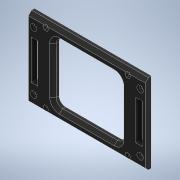
# Autodesk Inventor part: BottomHolder
Saved by Autodesk Inventor 2021 (Build 250183000, 183)
## iProperties
Created: 2020-11-06
Part Number: BottomHolder
Material: Generic
Document SubType Name: Modeling
Designer: lgnds
Density: 1 g/cm^3
Appearance: Default
Author: lgnds
Autodesk Inventor part; units mm, degrees
ref_plane "YZ Plane" through (0, 0, 0) normal (1, 0, 0) x (0, 1, 0)
ref_plane "XZ Plane" through (0, 0, 0) normal (0, 1, 0) x (-1, 0, 0)
ref_plane "XY Plane" through (0, 0, 0) normal (0, 0, 1) x (1, 0, 0)
sketch "Sketch1" plane through (0, 0, 0) normal (0, 0, 1) x (1, 0, 0)
  line L0 (-63.5, -54) -> (63.5, -54) construction
  line L1 (63.5, -54) -> (63.5, 54) construction
  line L2 (63.5, 54) -> (-63.5, 54) construction
  line L3 (-63.5, 54) -> (-63.5, -54) construction
  line L4 (-63.5, -54) -> (63.5, 54) construction
  line L5 (63.5, -54) -> (-63.5, 54) construction
  line L6 (-61.2483, 57.9) -> (-58.9967, 54) construction
  line L7 (-58.9967, 54) -> (-61.2483, 50.1) construction
  line L8 (-61.2483, 50.1) -> (-65.7517, 50.1) construction
  line L9 (-65.7517, 50.1) -> (-68.0033, 54) construction
  line L10 (-68.0033, 54) -> (-65.7517, 57.9) construction
  line L11 (-65.7517, 57.9) -> (-61.2483, 57.9) construction
  line L12 (-98.7, 0) -> (98.7, 0) construction
  line L13 (0, 86.8) -> (0, -86.8) construction
  line L14 (61.2483, 57.9) -> (58.9967, 54) construction
  line L15 (58.9967, 54) -> (61.2483, 50.1) construction
  line L16 (61.2483, 50.1) -> (65.7517, 50.1) construction
  line L17 (65.7517, 50.1) -> (68.0033, 54) construction
  line L18 (68.0033, 54) -> (65.7517, 57.9) construction
  line L19 (65.7517, 57.9) -> (61.2483, 57.9) construction
  line L20 (63.5, -54) -> (-63.5, -54) construction
  line L21 (-61.2483, -57.9) -> (-58.9967, -54) construction
  line L22 (-58.9967, -54) -> (-61.2483, -50.1) construction
  line L23 (-61.2483, -50.1) -> (-65.7517, -50.1) construction
  line L24 (-65.7517, -50.1) -> (-68.0033, -54) construction
  line L25 (-68.0033, -54) -> (-65.7517, -57.9) construction
  line L26 (-65.7517, -57.9) -> (-61.2483, -57.9) construction
  line L27 (61.2483, -57.9) -> (58.9967, -54) construction
  line L28 (58.9967, -54) -> (61.2483, -50.1) construction
  line L29 (61.2483, -50.1) -> (65.7517, -50.1) construction
  line L30 (65.7517, -50.1) -> (68.0033, -54) construction
  line L31 (68.0033, -54) -> (65.7517, -57.9) construction
  line L32 (65.7517, -57.9) -> (61.2483, -57.9) construction
  line L33 (-70.5, -62) -> (70.5, -62)
  line L34 (70.5, -62) -> (70.5, 62)
  line L35 (70.5, 62) -> (-70.5, 62)
  line L36 (-70.5, 62) -> (-70.5, -62)
  line L37 (-70.5, -62) -> (70.5, 62) construction
  line L38 (70.5, -62) -> (-70.5, 62) construction
  line L39 (-52.5, -46.1702) -> (52.5, -46.1702)
  line L40 (52.5, -46.1702) -> (52.5, 46.1702)
  line L41 (52.5, 46.1702) -> (-52.5, 46.1702)
  line L42 (-52.5, 46.1702) -> (-52.5, -46.1702)
  line L43 (-52.5, -46.1702) -> (52.5, 46.1702) construction
  line L44 (52.5, -46.1702) -> (-52.5, 46.1702) construction
  circle A0 centre (-63.5, 54) radius 2.4
  circle A1 centre (63.5, 54) radius 2.4
  circle A2 centre (63.5, -54) radius 2.4
  circle A3 centre (-63.5, -54) radius 2.4
  point P0 (0, 0)
  dimension "d0" = 7.8
  dimension "d1" = 127
  dimension "d2" = 108
  dimension "d3" = 124
  dimension "d4" = 141
  dimension "d5" = 18
  dimension "d8" = 4.8
  dimension "d9" = 4.8
  dimension "d10" = 4.8
  dimension "d11" = 4.8
  constraints: 86 end point, 21 symmetric about line, 8 coincident, 6 midpoint, 6 parallel, 4 centre point, 4 horizontal, 3 perpendicular, 1 point on line, 13 other
  measures "d0" distance between parallel lines of L8 L11
  measures "d1" distance of L1.end L2.end
  measures "d2" distance of L0.start L2.end
  measures "d3" distance between parallel lines of L33 L35
  measures "d4" distance between parallel lines of L34 L36
  measures "d5" distance between parallel lines of L36 L42
  measures "d8" diameter of A0
  measures "d9" diameter of A3
  measures "d10" diameter of A2
  measures "d11" diameter of A1
extrude "Extrusion1" add sketch "Sketch1" along normal blind 10
sketch "Sketch3" plane through (0, 0, 10) normal (0, 0, 1) x (1, 0, 0)
  circle A0 centre (-63.5, 54) radius 2.4 construction
  line L0 (-98.7, 0) -> (98.7, 0) construction
  line L1 (0, 86.8) -> (0, -86.8) construction
  line L2 (-61.2483, 57.9) -> (-58.9967, 54)
  line L3 (-58.9967, 54) -> (-61.2483, 50.1)
  line L4 (-61.2483, 50.1) -> (-65.7517, 50.1)
  line L5 (-65.7517, 50.1) -> (-68.0033, 54)
  line L6 (-68.0033, 54) -> (-65.7517, 57.9)
  line L7 (-65.7517, 57.9) -> (-61.2483, 57.9)
  circle A1 centre (63.5, 54) radius 2.4 construction
  line L8 (61.2483, 57.9) -> (58.9967, 54)
  line L9 (58.9967, 54) -> (61.2483, 50.1)
  line L10 (61.2483, 50.1) -> (65.7517, 50.1)
  line L11 (65.7517, 50.1) -> (68.0033, 54)
  line L12 (68.0033, 54) -> (65.7517, 57.9)
  line L13 (65.7517, 57.9) -> (61.2483, 57.9)
  circle A2 centre (-63.5, -54) radius 2.4 construction
  line L14 (-61.2483, -57.9) -> (-58.9967, -54)
  line L15 (-58.9967, -54) -> (-61.2483, -50.1)
  line L16 (-61.2483, -50.1) -> (-65.7517, -50.1)
  line L17 (-65.7517, -50.1) -> (-68.0033, -54)
  line L18 (-68.0033, -54) -> (-65.7517, -57.9)
  line L19 (-65.7517, -57.9) -> (-61.2483, -57.9)
  circle A3 centre (63.5, -54) radius 2.4 construction
  line L20 (61.2483, -57.9) -> (58.9967, -54)
  line L21 (58.9967, -54) -> (61.2483, -50.1)
  line L22 (61.2483, -50.1) -> (65.7517, -50.1)
  line L23 (65.7517, -50.1) -> (68.0033, -54)
  line L24 (68.0033, -54) -> (65.7517, -57.9)
  line L25 (65.7517, -57.9) -> (61.2483, -57.9)
  point P0 (0, 0)
  dimension "d12" = 7.8
  constraints: 48 end point, 24 symmetric about line, 4 coincident, 3 centre point, 1 horizontal, 16 other
  measures "d12" distance between parallel lines of L4 L7
extrude "Extrusion2" cut sketch "Sketch3" against normal blind 4
fillet "Fillet1" radius 10 4 edges at (-52.5, 46.1702, 5) (52.5, 46.1702, 5) (52.5, -46.1702, 5) (-52.5, -46.1702, 5)
chamfer "Chamfer1" distance 5 angle 45 8 edges at (0, 46.1702, 10) (49.5711, 43.2413, 10) (52.5, 0, 10) (49.5711, -43.2413, 10) (0, -46.1702, 10) (-49.5711, -43.2413, 10) (-52.5, 0, 10) (-49.5711, 43.2413, 10)
sketch "Sketch4" plane through (0, 0, 10) normal (0, 0, 1) x (1, 0, 0)
  line L0 (-70.5, -62) -> (70.5, -62) projected
  line L1 (-70.5, 62) -> (-90.5, 62)
  line L2 (-90.5, 62) -> (-90.5, -62)
  line L3 (-90.5, -62) -> (-70.5, -62)
  line L4 (-70.5, -62) -> (-70.5, 62)
  line L5 (0, 86.8) -> (0, -86.8) projected
  line L6 (70.5, 62) -> (90.5, 62)
  line L7 (90.5, 62) -> (90.5, -62)
  line L8 (90.5, -62) -> (70.5, -62)
  line L9 (70.5, -62) -> (70.5, 62)
  line L10 (-82.5, 62) -> (-82.5, -62) construction
  line L11 (-85.5, -30) -> (-79.5, -30)
  line L12 (-79.5, -30) -> (-79.5, 30)
  line L13 (-79.5, 30) -> (-85.5, 30)
  line L14 (-85.5, 30) -> (-85.5, -30)
  line L15 (-85.5, -30) -> (-79.5, 30) construction
  line L16 (-79.5, -30) -> (-85.5, 30) construction
  line L17 (82.5, 62) -> (82.5, -62) construction
  line L18 (85.5, -30) -> (79.5, -30)
  line L19 (79.5, -30) -> (79.5, 30)
  line L20 (79.5, 30) -> (85.5, 30)
  line L21 (85.5, 30) -> (85.5, -30)
  line L22 (85.5, -30) -> (79.5, 30) construction
  line L23 (79.5, -30) -> (85.5, 30) construction
  point P0 (0, 0)
  point P1 (-80.5, -62)
  point P2 (70.5, -62)
  point P3 (80.5, -62)
  point P4 (-82.5, 0)
  point P5 (82.5, 0)
  dimension "d19" = 20
  dimension "d25" = 8
  dimension "d26" = 6
  dimension "d27" = 60
  constraints: 44 end point, 13 symmetric about line, 6 midpoint, 4 parallel, 3 perpendicular, 3 point on line, 2 horizontal
  measures "d19" distance between parallel lines of L4 L2
  measures "d25" distance between parallel lines of L2 L10
  measures "d26" distance between parallel lines of L12 L14
  measures "d27" distance between parallel lines of L11 L13
extrude "Extrusion3" add sketch "Sketch4" against normal up to surface (10 mm away)
chamfer "Chamfer2" distance 5 angle 45 2 edges at (0, 62, 10) (0, -62, 10)
sketch "Sketch5" plane through (0, 0, 10) normal (0, 0, 1) x (1, 0, 0)
  line L0 (-85.5, -30) -> (-85.5, 30) construction
  line L1 (-79.5, 30) -> (-79.5, -30) construction
  line L2 (0, 86.8) -> (0, -86.8) projected
  line L3 (-82.5, 46.5549) -> (-82.5, -47.9965) construction
  circle A0 centre (-82.5, 45) radius 2.4
  circle A1 centre (-82.5, -45) radius 2.4
  line L4 (85.5, -30) -> (85.5, 30) construction
  line L5 (79.5, 30) -> (79.5, -30) construction
  line L6 (82.5, 46.5549) -> (82.5, -47.9965) construction
  circle A2 centre (82.5, 45) radius 2.4
  circle A3 centre (82.5, -45) radius 2.4
  point P0 (0, 0)
  dimension "d28" = 3
  dimension "d29" = 6
  dimension "d30" = 90
  dimension "d31" = 60
  dimension "d32" = 15
  dimension "d33" = 4.8
  dimension "d34" = 4.8
  constraints: 8 end point, 8 symmetric about line, 4 centre point, 4 point on line, 1 vertical, 2 other
  measures "d28" distance between parallel lines of L0 L3
  measures "d29" distance between parallel lines of L0 L1
  measures "d30" distance of A0.centre A1.centre
  measures "d31" distance of L1.end L1.start
  measures "d32" vertical distance of A1.centre L1.end
  measures "d33" diameter of A0
  measures "d34" diameter of A1
extrude "Extrusion4" cut sketch "Sketch5" against normal through all
sketch "Sketch6" plane through (0, 0, 10) normal (0, 0, 1) x (1, 0, 0)
  circle A0 centre (-82.5, 45) radius 2.4 projected
  circle A1 centre (-82.5, -45) radius 2.4 projected
  circle A2 centre (82.5, -45) radius 2.4 projected
  circle A3 centre (82.5, 45) radius 2.4 projected
  circle A4 centre (-82.5, 45) radius 5
  circle A5 centre (-82.5, -45) radius 5
  circle A6 centre (82.5, -45) radius 5
  circle A7 centre (82.5, 45) radius 5
  point P0 (0, 0)
  dimension "d37" = 10
  dimension "d38" = 10
  dimension "d39" = 10
  dimension "d40" = 10
  constraints: 4 centre point
  measures "d37" diameter of A4
  measures "d38" diameter of A5
  measures "d39" diameter of A7
  measures "d40" diameter of A6
extrude "Extrusion5" cut sketch "Sketch6" against normal blind 4 contours A0 | A1 | A2 | A3 | A4 | A5 | A6 | A7
sketch "Sketch7" plane through (0, 0, 10) normal (0, 0, 1) x (1, 0, 0)
  line L0 (-85.5, 30) -> (-79.5, 30) projected
  line L1 (-85.5, -30) -> (-85.5, 30) projected
  line L2 (-79.5, 30) -> (-79.5, -30) projected
  line L3 (-79.5, -30) -> (-85.5, -30) projected
  line L4 (79.5, -30) -> (79.5, 30) projected
  line L5 (79.5, 30) -> (85.5, 30) projected
  line L6 (85.5, 30) -> (85.5, -30) projected
  line L7 (85.5, -30) -> (79.5, -30) projected
  line L8 (-79, 30.5) -> (-86, 30.5)
  line L9 (-86, 30.5) -> (-86, -30.5)
  line L10 (-86, -30.5) -> (-79, -30.5)
  line L11 (-79, -30.5) -> (-79, 30.5)
  line L12 (86, 30.5) -> (79, 30.5)
  line L13 (79, 30.5) -> (79, -30.5)
  line L14 (79, -30.5) -> (86, -30.5)
  line L15 (86, -30.5) -> (86, 30.5)
  point P0 (0, 0)
  dimension "d43" = 0.5
  dimension "d44" = 0.5
  constraints: 16 end point, 6 other
  measures "d43" distance between parallel lines of L8 L0
  measures "d44" distance between parallel lines of L12 L5
extrude "Extrusion6" cut sketch "Sketch7" against normal through all
thicken "Thicken1" operation add thickness 3 both sides no extend neighbours yes toward (-1, 0, 0) faces at (79, 10.1667, 6.6667)
thicken "Thicken2" operation add thickness 3 both sides no extend neighbours yes toward (1, 0, 0) faces at (-79, 10.1667, 3.3333)
chamfer "Chamfer3" distance 0.5 angle 45 28 edges at (0, -62, 0) (-90.5, 0, 0) (0, 62, 0) (90.5, 0, 0) (86, 0, 0) (81, 30.5, 0) (76, 0, 0) (81, -30.5, 0) (80.1, -45, 0) (61.1, -54, 0) (61.1, 54, 0) (80.1, 45, 0) (-65.9, 54, 0) (-84.9, 45, 0) (-81, 30.5, 0) (-76, 0, 0) (-86, 0, 0) (-81, -30.5, 0) (-84.9, -45, 0) (-65.9, -54, 0) (-49.5711, -43.2413, 0) (-52.5, 0, 0) (-49.5711, 43.2413, 0) (0, 46.1702, 0) (49.5711, 43.2413, 0) (52.5, 0, 0) (49.5711, -43.2413, 0) (0, -46.1702, 0)
equation "\"d9\" = d8"
equation "\"d10\" = d9"
equation "\"d11\" = d8"
equation "\"d28\" = 0.5 * d29"
equation "\"d32\" = -0.5 * d31 + 0.5 * d30"
equation "\"d34\" = d33"
equation "\"d38\" = d37"
equation "\"d39\" = d37"
equation "\"d40\" = d38"
body "Solid1"
